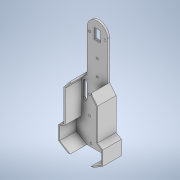
# Autodesk Inventor part: Top_Lid
Saved by Autodesk Inventor 2021 (Build 250183000, 183)
## iProperties
Created: 2024-05-18
Part Number: Top_Lid
Material: Generic
Document SubType Name: Modeling
Designer: Lukas
Density: 1 g/cm^3
Appearance: Default
Author: Lukas
Autodesk Inventor part; units mm, degrees
ref_plane "YZ Plane" through (0, 0, 0) normal (1, 0, 0) x (0, 1, 0)
ref_plane "XZ Plane" through (0, 0, 0) normal (0, 1, 0) x (-1, 0, 0)
ref_plane "XY Plane" through (0, 0, 0) normal (0, 0, 1) x (1, 0, 0)
sketch "Sketch1" plane through (0, 0, 0) normal (0, 0, 1) x (1, 0, 0)
  line L0 (16, 59.6) -> (16, -59.6)
  line L1 (16, -59.6) -> (-16, -59.6)
  line L2 (-16, -59.6) -> (-16, 59.6)
  arc A0 (16, 59.6) -> (-16, 59.6) centre (0, 59.6) ccw
  circle A1 centre (12, 55.6) radius 1.6
  circle A2 centre (-12, 55.6) radius 1.6
  circle A3 centre (12, -29.6) radius 1.6
  circle A4 centre (12, -58.6) radius 1.6
  circle A5 centre (-12, -29.6) radius 1.6
  circle A6 centre (-12, -58.6) radius 1.6
  line L3 (-16, -59.6) -> (-32.5, -69.6)
  line L4 (-32.5, -69.6) -> (-32.5, -89.6)
  line L5 (-32.5, -89.6) -> (-16, -99.6)
  line L6 (-16, -99.6) -> (16, -99.6)
  line L7 (16, -99.6) -> (32.5, -89.6)
  line L8 (32.5, -89.6) -> (32.5, -69.6)
  line L9 (32.5, -69.6) -> (16, -59.6)
  line L10 (-5, 64.6) -> (5, 64.6)
  line L11 (5, 64.6) -> (5, 48.6)
  line L12 (5, 48.6) -> (-5, 48.6)
  line L13 (-5, 48.6) -> (-5, 64.6)
  circle A7 centre (0, 25) radius 1.4
  circle A8 centre (0, 0) radius 1.4
  circle A9 centre (10, -94.6) radius 1.4
  circle A10 centre (-10, -94.6) radius 1.4
  point P0 (0, -59.6)
  point P1 (-16, 0)
  point P2 (-13.249, -59.6)
  point P3 (-10.751, -59.6)
  point P4 (10.751, -59.6)
  point P5 (13.249, -59.6)
  point P6 (0, -99.6)
  point P7 (0, 48.6)
  dimension "d0" = 32
  dimension "d1" = 119.2
  dimension "d4" = 4
  dimension "d5" = 12
  dimension "d6" = 12
  dimension "d7" = 3.2
  dimension "d8" = 85.2
  dimension "d9" = 29
  dimension "d10" = 10
  dimension "d11" = 10
  dimension "d12" = 16.5
  dimension "d13" = 16.5
  dimension "d14" = 40
  dimension "d54" = 10
  dimension "d55" = 11
  dimension "d56" = 16
  dimension "d57" = 2.8
  dimension "d58" = 25
  dimension "d59" = 2.8
  dimension "d60" = 35
  dimension "d61" = 10
  dimension "d62" = 10
  constraints: 28 end point, 11 centre point, 8 vertical alignment, 7 equal radius, 5 horizontal alignment, 5 perpendicular, 4 midpoint, 3 equal length, 2 parallel, 2 point on circle, 2 tangent, 2 vertical, 1 coincident, 1 horizontal
  measures "d0" distance of L0.end L1.end
  measures "d1" distance of L0.start L0.end
  measures "d4" vertical distance of A1.centre A0.centre
  measures "d5" horizontal distance of A0.centre A1.centre
  measures "d6" horizontal distance of A2.centre A0.centre
  measures "d7" diameter of A1
  measures "d8" distance of A3.centre A1.centre
  measures "d9" distance of A4.centre A3.centre
  measures "d10" vertical distance of L4.end L5.end
  measures "d11" vertical distance of L1.end L3.end
  measures "d12" horizontal distance of L1.end L3.end
  measures "d13" horizontal distance of L4.end L5.end
  measures "d14" distance between parallel lines of L6 L1
  measures "d54" distance of L11.end L12.end
  measures "d55" distance from line of A0.centre L12
  measures "d56" distance of L12.end L10.start
  measures "d57" diameter of A7
  measures "d58" distance of A7.centre point (0, 0)
  measures "d59" diameter of A9
  measures "d60" distance from line of L1 A9.centre
  measures "d61" horizontal distance of A10.centre point (0, -99.6)
  measures "d62" horizontal distance of A9.centre point (0, -99.6)
extrude "Extrusion1" add sketch "Sketch1" along normal blind 3 contours L0 L1 A4 A6 L2 A0 | L9 L8 L7 L6 L5 L4 L3 L1 A6 A4
sketch "Sketch2" plane through (0, 0, 0) normal (0, 0, -1) x (-1, 0, 0)
  circle A0 centre (12, -58.6) radius 1.6 projected
  circle A1 centre (-12, 55.6) radius 1.6 projected
  circle A2 centre (12, 55.6) radius 1.6 projected
  circle A3 centre (-12, -29.6) radius 1.6 projected
  circle A4 centre (12, -29.6) radius 1.6 projected
  circle A5 centre (-12, -58.6) radius 1.6 projected
  line L0 (-16, -59.6) -> (-16, 59.6) projected
  line L1 (-32.5, -69.6) -> (-16, -59.6) projected
  line L2 (-32.5, -89.6) -> (-32.5, -69.6) projected
  line L3 (-16, -99.6) -> (-32.5, -89.6) projected
  line L4 (16, -99.6) -> (-16, -99.6) projected
  line L5 (32.5, -89.6) -> (16, -99.6) projected
  line L6 (32.5, -69.6) -> (32.5, -89.6) projected
  line L7 (16, -59.6) -> (32.5, -69.6) projected
  line L8 (16, 59.6) -> (16, -59.6) projected
  arc A6 (16, 59.6) -> (-16, 59.6) centre (0, 59.6) ccw projected
  line L9 (-16, -59.6) -> (-16, 59.6) projected
  line L10 (-16, -57.2614) -> (-34.5, -68.4735)
  line L11 (-34.5, -68.4735) -> (-34.5, -90.7265)
  line L12 (-34.5, -90.7265) -> (-19.8588, -99.6)
  line L13 (16, -99.6) -> (-16, -99.6) projected
  line L14 (-19.8588, -99.6) -> (-16, -99.6)
  line L15 (32.5, -89.6) -> (16, -99.6) projected
  line L16 (16, -99.6) -> (19.8588, -99.6)
  line L17 (19.8588, -99.6) -> (34.5, -90.7265)
  line L18 (34.5, -90.7265) -> (34.5, -68.4735)
  line L19 (34.5, -68.4735) -> (16, -57.2614)
  line L20 (16, 59.6) -> (16, -59.6) projected
  line L21 (16, -59.6) -> (32.5, -69.6) projected
  line L22 (-32.5, -69.6) -> (-16, -59.6) projected
  line L23 (16.3859, -99.6) -> (32.7, -89.7127)
  line L24 (32.7, -89.7127) -> (32.7, -69.4873)
  line L25 (32.7, -69.4873) -> (24.2, -64.3358)
  line L26 (-16, -99.6) -> (-32.5, -89.6) projected
  line L27 (-32.5, -89.6) -> (-32.5, -69.6) projected
  line L28 (-16.3859, -99.6) -> (-32.7, -89.7127)
  line L29 (-32.7, -89.7127) -> (-32.7, -69.4873)
  line L30 (-32.7, -69.4873) -> (-24.2, -64.3358)
  line L31 (32.5, -69.6) -> (32.5, -89.6) projected
  line L32 (24.2, -64.3358) -> (24.2, -62.2311)
  line L33 (-24.2, -64.3358) -> (-24.2, -62.2311)
  point P0 (0, 0)
  point P1 (16, -59.2661)
  point P2 (-16, -59.2661)
  dimension "d15" = 2
  dimension "d16" = 2
  dimension "d17" = 2
  dimension "d18" = 2
  dimension "d19" = 2
  dimension "d20" = 2
  dimension "d26" = 0.2
  dimension "d27" = 0.2
  dimension "d28" = 0.2
  dimension "d29" = 0.2
  dimension "d30" = 0.2
  dimension "d31" = 0.2
  dimension "d34" = 8.2
  dimension "d35" = 8.2
  constraints: 32 end point, 12 parallel, 6 point on line, 4 vertical, 1 collinear, 1 horizontal, 1 perpendicular
  measures "d15" distance between parallel lines of L19 L7
  measures "d16" distance between parallel lines of L6 L18
  measures "d17" distance between parallel lines of L5 L17
  measures "d18" distance between parallel lines of L12 L3
  measures "d19" distance between parallel lines of L11 L2
  measures "d20" distance between parallel lines of L10 L1
  measures "d26" distance between parallel lines of L3 L28
  measures "d27" distance between parallel lines of L29 L27
  measures "d28" distance between parallel lines of L30 L1
  measures "d29" distance between parallel lines of L5 L23
  measures "d30" distance between parallel lines of L6 L24
  measures "d31" distance between parallel lines of L7 L25
  measures "d34" distance between parallel lines of L32 L8
  measures "d35" distance between parallel lines of L0 L33
extrude "Extrusion2" add sketch "Sketch2" against normal blind 29 contours L33 L30 L29 L28 L14 L12 L11 L10 | L19 L18 L17 L16 L23 L24 L25 L32
extrude "Extrusion3" add sketch "Sketch2" against normal up to surface (3 mm away) contours L1 L2 L3 L14 L28 L29 L30 L33 L10 L0 | L19 L32 L25 L24 L23 L16 L5 L6 L7 L8
sketch "Sketch3" plane through (0, 0, 0) normal (0, 0, -1) x (-1, 0, 0)
  line L0 (-16, -57.2614) -> (-34.5, -68.4735) projected
  line L1 (-16, -57.2614) -> (-16, 59.6) projected
  line L2 (16, 59.6) -> (16, -57.2614) projected
  line L3 (34.5, -68.4735) -> (16, -57.2614) projected
  line L4 (-26.2, -63.4432) -> (-26.2, -13.6343)
  line L5 (-26.2, -13.6343) -> (-16, -0.8843)
  line L6 (26.2, -63.4432) -> (26.2, -13.6343)
  line L7 (26.2, -13.6343) -> (16, -0.8843)
  line L8 (-24.2, -62.2311) -> (-24.2, -64.3358) projected
  line L9 (24.2, -64.3358) -> (24.2, -62.2311) projected
  line L10 (-24.2, -62.2311) -> (-24.2, -14.3358)
  line L11 (-24.2, -14.3358) -> (-16, -4.0858)
  line L12 (-16, -57.2614) -> (-16, 59.6) projected
  line L13 (24.2, -62.2311) -> (24.2, -14.3358)
  line L14 (24.2, -14.3358) -> (16, -4.0858)
  line L15 (-16.2, -4.3358) -> (-16.2, -1.1343)
  line L16 (16.2, -4.3358) -> (16.2, -1.1343)
  line L17 (19, -16.0858) -> (19, -38.0858) construction
  line L18 (16, -16.0858) -> (16, -38.0858)
  line L19 (22, -38.0858) -> (22, -16.0858)
  arc A0 (22, -16.0858) -> (16, -16.0858) centre (19, -16.0858) ccw
  arc A1 (16, -38.0858) -> (22, -38.0858) centre (19, -38.0858) ccw
  line L20 (-19, -16.0858) -> (-19, -38.0858) construction
  line L21 (-22, -16.0858) -> (-22, -38.0858)
  line L22 (-16, -38.0858) -> (-16, -16.0858)
  arc A2 (-16, -16.0858) -> (-22, -16.0858) centre (-19, -16.0858) ccw
  arc A3 (-22, -38.0858) -> (-16, -38.0858) centre (-19, -38.0858) ccw
  point P0 (0, 0)
  point P1 (19, -27.0858)
  point P2 (-19, -27.0858)
  point P3 (-20.1, -9.2108)
  dimension "d36" = 2
  dimension "d37" = 2
  dimension "d39" = 2
  dimension "d46" = 50
  dimension "d47" = 0.2
  dimension "d48" = 0.2
  dimension "d49" = 10
  dimension "d50" = 6
  dimension "d52" = 22
  dimension "d53" = 12
  constraints: 36 end point, 13 point on line, 8 point on circle, 8 tangent, 6 parallel, 5 vertical, 4 centre point, 4 horizontal alignment, 3 midpoint, 1 equal length, 1 equal radius
  measures "d36" distance between parallel lines of L6 L13
  measures "d37" distance between parallel lines of L4 L10
  measures "d39" distance between parallel lines of L7 L14
  measures "d46" distance of L9.start L13.end
  measures "d47" distance between parallel lines of L2 L16
  measures "d48" distance between parallel lines of L15 L12
  measures "d49" vertical distance of L16.start L13.end
  measures "d50" distance between parallel lines of L18 L19
  measures "d52" distance of L17.start L17.end
  measures "d53" vertical distance of L14.end L17.start
extrude "Extrusion4" add sketch "Sketch3" against normal up to surface (3 mm away) contours L0 L10 L11 L1 A2 L21 A3 | L0 L4 L5 L15 L11 L10 | L15 L5 L1 L11 | L7 L16 L14 L2 | L14 L13 L3 L2 A1 L19 A0 | L7 L6 L3 L13 L14 L16
extrude "Extrusion5" add sketch "Sketch3" against normal up to surface (29 mm away) contours L0 L4 L5 L15 L11 L10 | L7 L6 L3 L13 L14 L16
equation "\"d6\" = d5"
equation "\"d13\" = d12"
equation "\"d62\" = d61"
equation "\"d16\" = d15"
equation "\"d17\" = d16"
equation "\"d18\" = d17"
equation "\"d19\" = d18"
equation "\"d20\" = d19"
equation "\"d27\" = d26"
equation "\"d28\" = d27"
equation "\"d29\" = d26"
equation "\"d30\" = d29"
equation "\"d31\" = d30"
equation "\"d34\" = d35"
equation "\"d37\" = d36"
body "Solid1"
